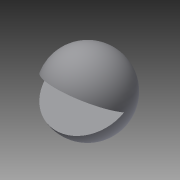
# Autodesk Inventor part: Pacman2
Saved by Autodesk Inventor 2015 (Build 190159000, 159)
## iProperties
Created: 2015-04-11
Part Number: Pacman2
Material: Generic
Document SubType Name: Modeling
Designer: tquinn
Density: 1 g/cm^3
Appearance: Default
Author: tquinn
Autodesk Inventor part; units mm, degrees
ref_plane "YZ Plane" through (0, 0, 0) normal (1, 0, 0) x (0, 1, 0)
ref_plane "XZ Plane" through (0, 0, 0) normal (0, 1, 0) x (-1, 0, 0)
ref_plane "XY Plane" through (0, 0, 0) normal (0, 0, 1) x (1, 0, 0)
sketch "Sketch1" plane through (0, 0, 0) normal (0, 0, 1) x (1, 0, 0)
  circle A0 centre (0, 0) radius 13.97
  line L0 (0, 13.97) -> (0, -13.97)
  dimension "d0" = 27.94
  constraints: 2 end point, 2 point on circle, 1 centre point, 1 coincident, 1 vertical
  measures "d0" diameter of A0
revolve "Revolution1" add sketch "Sketch1" angle 360 about axis through (0, 13.97, 0) along (0, -1, 0) picked at (-7.7107, -1.7324) contours L0 A0
sketch "Sketch3" plane through (0, 0, 0) normal (1, 0, 0) x (0, 1, 0)
  circle A0 centre (0, 0) radius 13.97 projected
  line L0 (0, 0) -> (0, 13.97)
  line L1 (0, 0) -> (6.985, 12.0984)
  line L2 (0, 0) -> (-6.985, 12.0984)
  dimension "d2" = 30
  dimension "d3" = 30
  constraints: 6 end point, 3 point on circle, 1 vertical
  measures "d2" angle of L0 L1
  measures "d3" angle of L2 L0
extrude "Extrusion1" cut sketch "Sketch3" along normal mid plane 50.8 contours L1 L0 A0 | A0 L0 L2
equation "\"d3\" = d2"
body "Solid1"
